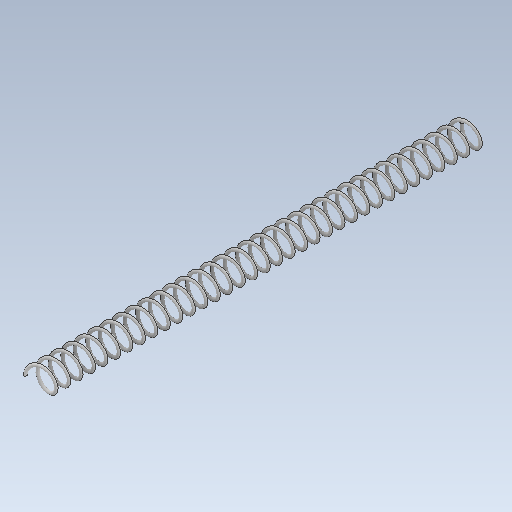
# Autodesk Inventor part: LOC0014
Saved by Autodesk Inventor 2020 (Build 240168000, 168)
## iProperties
Created: 2021-01-30
Part Number: LOC0014
Material: Generic
Document SubType Name: Modeling
Designer: kishore.balu
Density: 1 g/cm^3
Appearance: Default
Description: Spring
Engineer: LOKESH BABU/SRI SAI
Author: LOKESH BABU/SRI SAI
Title: MABC-N
Autodesk Inventor part; units mm, degrees
ref_plane "YZ Plane" through (0, 0, 0) normal (1, 0, 0) x (0, 1, 0)
ref_plane "XZ Plane" through (0, 0, 0) normal (0, 1, 0) x (-1, 0, 0)
ref_plane "XY Plane" through (0, 0, 0) normal (0, 0, 1) x (1, 0, 0)
sketch "Sketch1" plane through (0, 0, 0) normal (0, 1, 0) x (-1, 0, 0)
  line L0 (0, 0) -> (0, -35)
  dimension "d0" = 35
  constraints: 2 end point, 1 vertical
  measures "d0" distance of L0.start L0.end
sketch "Sketch2" plane through (0, 0, 0) normal (0, 1, 0) x (-1, 0, 0)
  circle A0 centre (1, 0) radius 0.125
  point P0 (0, 0)
  dimension "d1" = 0.25
  dimension "d2" = 1
  constraints: 1 centre point
  measures "d1" diameter of A0
  measures "d2" distance of A0.centre point (0, 0)
coil "Coil1" sketch "Sketch2" operation add axis through (0, 0, 0) along (0, 0, -1) pitch 1 turns 35 hand right
body "Solid1"
